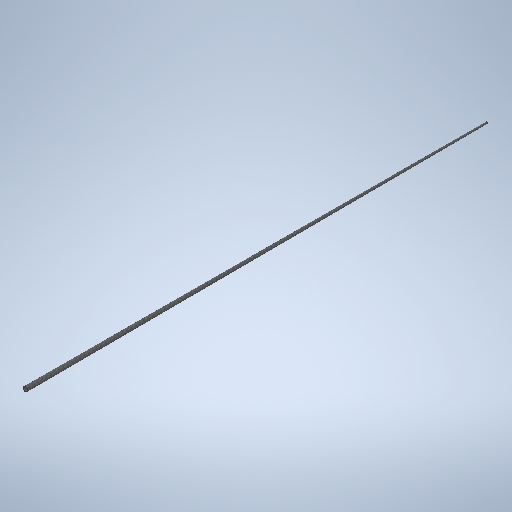
# Autodesk Inventor part: Rear Wing Spar (tapered hollow)
Saved by Autodesk Inventor 2025.1 (Build 291241000, 241)
## iProperties
Created: 2025-01-29
Part Number: Rear Wing Spar (tapered hollow)
Material: CFRP
Document SubType Name: Modeling
Designer: chowg
Density: 1.43 g/cm^3
Appearance: Carbon Fiber
Category: <PART CATAGORY>
Title: <TITLE>
Author: chowg
Revision Number: 1
Autodesk Inventor part; units mm, degrees
ref_plane "YZ Plane" through (0, 0, 0) normal (1, 0, 0) x (0, 1, 0)
ref_plane "XZ Plane" through (0, 0, 0) normal (0, 1, 0) x (-1, 0, 0)
ref_plane "XY Plane" through (0, 0, 0) normal (0, 0, 1) x (1, 0, 0)
sketch "Sketch6" plane through (0, 0, 0) normal (1, 0, 0) x (0, 1, 0)
  line L0 (0, 0) -> (6.225, 0) construction
  line L1 (6.225, 0) -> (6.625, 0)
  line L2 (0, 0) -> (0, -2.5827)
  line L3 (0, 0) -> (2.5827, 0) construction
  line L4 (2.1, -1320) -> (6.225, 0)
  line L5 (2.1, -1320) -> (2.5, -1320)
  line L6 (2.1, -1320) -> (2.5, -1320) construction
  line L7 (2.5, -1320) -> (6.625, 0)
  dimension "d85" = 6.225
  dimension "d87" = 0.4
  dimension "d89" = 90
  dimension "d93" = 0.4
  dimension "d94" = 0
  constraints: 16 end point, 4 horizontal, 2 equal length, 1 parallel
  measures "d85" distance of L0.start L1.start
  measures "d87" distance of L1.start L1.end
  measures "d89" angle of L2 L3
  measures "d93" distance of L4.start L5.end
  measures "d94" distance between parallel lines of L5 L6
revolve "Revolution1" add sketch "Sketch6" angle 360 about axis through (0, 0, 0) along (0, 0, -1)
body "Solid2"
